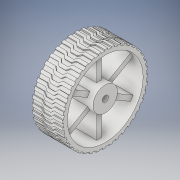
# Autodesk Inventor part: wheel
Saved by Autodesk Inventor 2019 (Build 230136000, 136)
## iProperties
Created: 2020-12-06
Part Number: wheel
Material: Пластик АБС
Document SubType Name: Modeling
Designer: Professional
Density: 1.06 g/cm^3
Appearance: Гладкий — белый
Author: Professional
Autodesk Inventor part; units mm, degrees
ref_plane "YZ Plane" through (0, 0, 0) normal (1, 0, 0) x (0, 1, 0)
ref_plane "XZ Plane" through (0, 0, 0) normal (0, 1, 0) x (-1, 0, 0)
sketch "Эскиз1" plane through (0, 0, 0) normal (1, 0, 0) x (0, 1, 0)
  circle A0 centre (0, 0) radius 35
  circle A1 centre (0, 0) radius 31
  circle A2 centre (0, 0) radius 10
  circle A3 centre (0, 0) radius 2.5
  dimension "d0" = 70
  dimension "d1" = 4
  dimension "d2" = 20
  dimension "d3" = 5
  constraints: 4 centre point, 4 coincident
  measures "d0" diameter of A0
  measures "d1" radial gap between concentric circles of A0 A1
  measures "d2" diameter of A2
  measures "d3" diameter of A3
extrude "Выдавливание1" add sketch "Эскиз1" along normal blind 25
sketch "Эскиз2" plane through (0, 0, 0) normal (-1, 0, 0) x (0, 0, 1)
  circle A0 centre (0, 0) radius 10 projected
  line L0 (-2, -9.798) -> (-2, -30.9354)
  circle A1 centre (0, 0) radius 31 projected
  line L1 (2, -9.798) -> (2, -30.9354)
  dimension "d6" = 4
  constraints: 4 end point, 4 point on circle, 2 vertical, 1 parallel
  measures "d6" distance between parallel lines of L0 L1
extrude "Выдавливание2" add sketch "Эскиз2" against normal blind 20 contours A0 L1 A1 L0 picked at (-0.2224, -16.9826)
pattern_circular "Круговой массив1" count 6 over 360 about axis through (0, 0, 0) along (1, 0, 0) of "Выдавливание2"
ref_plane "РабПлоскость1" through (0, 30.3109, 17.5) normal (0, 0.866, 0.5) x (-1, 0, 0)
sketch "Эскиз3" plane through (0, 30.3109, 17.5) normal (0, 0.866, 0.5) x (-1, 0, 0)
  line L0 (-25, 10) -> (-25, -10) projected
  line L1 (-25, 1.5) -> (-17.5, 1.5)
  line L2 (0, 6.631) -> (-20, 6.631) projected
  line L3 (-17.5, 1.5) -> (-15.1861, 3.8139)
  line L4 (-15.1861, 3.8139) -> (-9.8139, 3.8139)
  line L5 (-9.8139, 3.8139) -> (-7.5, 1.5)
  line L6 (-7.5, 1.5) -> (0, 1.5)
  line L7 (0, 1.5) -> (0, -1.5)
  line L8 (0, -1.5) -> (-7.5, -1.5)
  line L9 (-7.5, -1.5) -> (-9.8139, 0.8139)
  line L10 (-9.8139, 0.8139) -> (-15.1861, 0.8139)
  line L11 (-15.1861, 0.8139) -> (-17.5, -1.5)
  line L12 (-17.5, -1.5) -> (-25, -1.5)
  line L13 (0, -35) -> (0, 35) projected
  line L14 (-25, 1.5) -> (-25, -1.5)
  point P0 (0, 0)
  point P1 (0, 0)
  dimension "d12" = 2.3139
  dimension "d13" = 3
  dimension "d14" = 10
  constraints: 24 end point, 7 equal length, 6 point on line, 4 perpendicular, 3 parallel, 2 midpoint, 1 collinear
  measures "d12" distance between parallel lines of L6 L4
  measures "d13" distance between parallel lines of L6 L8
  measures "d14" distance of L8.end L11.end
extrude "Выдавливание3" cut sketch "Эскиз3" against normal blind 1
pattern_circular "Круговой массив2" count 40 over 360 about axis through (0, 0, 0) along (1, 0, 0) of "Выдавливание3"
